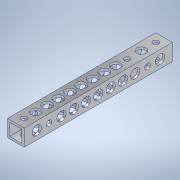
# Autodesk Inventor part: 上下直動9x9_1_CPY
Saved by Autodesk Inventor 2020.3 (Build 243373000, 373)
## iProperties
Created: 2020-07-05
Part Number: 上下直動9x9_1_CPY
Material: アルミニウム 6061
Document SubType Name: Modeling
Designer: totot
Mass: 7.85802 g
Surface Area: 50.3861 cm^2
Volume: 2.91038 cm^3
Density: 2.7 g/cm^3
Appearance: アルミニウム - フラット
Author: totot
Autodesk Inventor part; units mm, degrees
ref_plane "YZ Plane" through (0, 0, 0) normal (1, 0, 0) x (0, 1, 0)
ref_plane "XZ Plane" through (0, 0, 0) normal (0, 1, 0) x (-1, 0, 0)
ref_plane "XY Plane" through (0, 0, 0) normal (0, 0, 1) x (1, 0, 0)
sketch "スケッチ1" plane through (0, 0, 0) normal (0, 0, 1) x (1, 0, 0)
  line L0 (0, 0) -> (9, 0)
  line L1 (9, 0) -> (9, -9)
  line L2 (9, -9) -> (0, -9)
  line L3 (0, -9) -> (0, 0)
  line L4 (1.2, -1.2) -> (7.8, -1.2)
  line L5 (7.8, -1.2) -> (7.8, -7.8)
  line L6 (7.8, -7.8) -> (1.2, -7.8)
  line L7 (1.2, -7.8) -> (1.2, -1.2)
  dimension "d0" = 9
  dimension "d1" = 9
  dimension "d2" = 6.6
  dimension "d3" = 6.6
  dimension "d4" = 1.2
  dimension "d5" = 1.2
  constraints: 16 end point, 4 parallel, 2 horizontal, 2 perpendicular
  measures "d0" distance of L1.end L2.end
  measures "d1" distance of L0.end L1.end
  measures "d2" distance of L5.end L6.end
  measures "d3" distance of L4.end L5.end
  measures "d4" distance between parallel lines of L3 L7
  measures "d5" distance between parallel lines of L4 L0
extrude "押し出し1" add sketch "スケッチ1" along normal blind 80
sketch "スケッチ3" plane through (0, -9, 0) normal (0, -1, 0) x (1, 0, 0)
  line L0 (0, 80) -> (9, 80) projected
  line L1 (0, 0) -> (9, 0) projected
  line L2 (9, 0) -> (9, 80) projected
  point P0 (4.5, 4.5)
  point P1 (4.5, 75.5)
  dimension "d20" = 4.5
  dimension "d21" = 4.5
  dimension "d22" = 4.5
  dimension "d23" = 4.5
  measures "d20" distance from line of point (4.5, 75.5) L0
  measures "d21" distance from line of L1 point (4.5, 4.5)
  measures "d22" distance from line of point (4.5, 4.5) L2
  measures "d23" distance from line of point (4.5, 75.5) L2
hole "穴2" at (4.5, -9, 4.5) at (4.5, -9, 75.5) direction (0, 1, 0) diameter 3 end through all
sketch "スケッチ4" plane through (9, -9, 0) normal (1, 0, 0) x (0, 0, -1)
  line L0 (0, 0) -> (0, 9) projected
  line L1 (-80, 0) -> (-80, 9) projected
  line L2 (0, 0) -> (-80, 0) projected
  point P0 (-13.5, 4.5)
  point P1 (-66.5, 4.5)
  dimension "d31" = 13.5
  dimension "d32" = 13.5
  dimension "d33" = 4.5
  dimension "d34" = 4.5
  measures "d31" distance from line of point (-13.5, 4.5) L0
  measures "d32" distance from line of point (-66.5, 4.5) L1
  measures "d33" distance from line of L2 point (-66.5, 4.5)
  measures "d34" distance from line of L2 point (-13.5, 4.5)
hole "穴3" at (9, -4.5, 13.5) at (9, -4.5, 66.5) direction (-1, 0, 0) diameter 3 end through all
sketch "スケッチ5" plane through (0, -9, 0) normal (0, -1, 0) x (1, 0, 0)
  line L0 (0, 0) -> (0, 80) projected
  line L1 (0, 0) -> (9, 0) projected
  point P0 (4.5, 20)
  dimension "d42" = 4.5
  dimension "d43" = 20
  measures "d42" distance from line of point (4.5, 20) L0
  measures "d43" distance from line of point (4.5, 20) L1
hole "穴4" at (4.5, -9, 20) direction (0, 1, 0) diameter 3 end through all
sketch "スケッチ6" plane through (0, -9, 0) normal (0, -1, 0) x (1, 0, 0)
  circle A0 centre (4.5, 4.5) radius 1.5 projected
  circle A1 centre (4.5, 75.5) radius 1.5 projected
  line L0 (4.5, 4.5) -> (4.5, 75.5)
  circle A2 centre (4.5, 20) radius 1.5 projected
  point P0 (0, 0)
  point P1 (4.5, 12.25)
  point P2 (4.5, 26.1667)
  point P3 (4.5, 32.3333)
  point P4 (4.5, 38.5)
  point P5 (4.5, 44.6667)
  point P6 (4.5, 50.8333)
  point P7 (4.5, 57)
  point P8 (4.5, 63.1667)
  point P9 (4.5, 69.3333)
  dimension "d51" = 15.5
  dimension "d52" = 7.75
  dimension "d53" = 55.5
  dimension "d54" = 6.1667
  dimension "d57" = 6.1667
  constraints: 2 end point, 2 point on line, 2 vertical, 7 other
  measures "d51" distance of L0.start A2.centre
  measures "d52" distance of point (4.5, 12.25) L0.start
  measures "d53" distance of L0.end A2.centre
  measures "d54" distance of point (4.5, 26.167) A2.centre
  measures "d57" distance of point (4.5, 26.167) point (4.5, 32.333)
hole "穴5" at (4.5, -9, 12.25) at (4.5, -9, 26.1667) at (4.5, -9, 32.3333) at (4.5, -9, 38.5) at (4.5, -9, 44.6667) at (4.5, -9, 50.8333) at (4.5, -9, 57) at (4.5, -9, 63.1667) at (4.5, -9, 69.3333) direction (0, 1, 0) diameter 5 end through all
sketch "スケッチ7" plane through (0, -9, 0) normal (-1, 0, 0) x (0, 0, 1)
  circle A0 centre (66.5, 4.5) radius 1.5 projected
  line L0 (80, 9) -> (80, 0) projected
  line L1 (0, 9) -> (80, 9) projected
  line L2 (0, 9) -> (0, 0) projected
  circle A1 centre (13.5, 4.5) radius 1.5 projected
  circle A2 centre (66.5, 4.5) radius 1.5 projected
  line L3 (13.5, 4.5) -> (66.5, 4.5)
  point P0 (6.75, 4.5)
  point P1 (73.25, 4.5)
  point P2 (20.125, 4.5)
  point P3 (26.75, 4.5)
  point P4 (33.375, 4.5)
  point P5 (40, 4.5)
  point P6 (46.625, 4.5)
  point P7 (53.25, 4.5)
  point P8 (59.875, 4.5)
  dimension "d69" = 6.75
  dimension "d70" = 13.5
  dimension "d71" = 4.5
  dimension "d72" = 6.75
  dimension "d73" = 4.5
  dimension "d74" = 53
  dimension "d75" = 6.625
  dimension "d78" = 6.625
  constraints: 2 end point, 2 horizontal, 1 point on line, 6 other
  measures "d69" distance of point (73.25, 4.5) A0.centre
  measures "d70" distance from line of L0 A0.centre
  measures "d71" distance from line of point (73.25, 4.5) L1
  measures "d72" distance from line of point (6.75, 4.5) L2
  measures "d73" distance from line of L1 point (6.75, 4.5)
  measures "d74" distance of A0.centre L3.start
  measures "d75" distance of point (20.125, 4.5) L3.start
  measures "d78" distance of point (20.125, 4.5) point (26.75, 4.5)
hole "穴6" at (0, -4.5, 6.75) at (0, -4.5, 73.25) at (0, -4.5, 20.125) at (0, -4.5, 26.75) at (0, -4.5, 33.375) at (0, -4.5, 40) at (0, -4.5, 46.625) at (0, -4.5, 53.25) at (0, -4.5, 59.875) direction (1, 0, 0) diameter 5 end through all
equation "\"d22\" = d21"
equation "\"d23\" = d20"
equation "\"d32\" = d31"
equation "\"d34\" = d33"
equation "\"d52\" = 0.5 * d51"
equation "\"d54\" = 0.111111 * d53"
equation "\"d57\" = d54"
equation "\"d69\" = 0.5 * d70"
equation "\"d72\" = d69"
equation "\"d75\" = 0.125 * d74"
equation "\"d78\" = d75"
